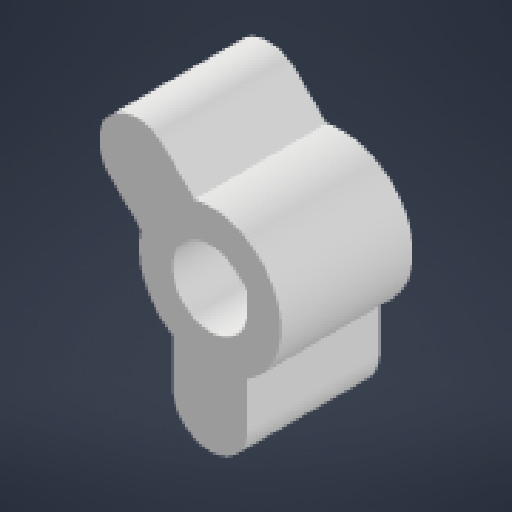
# Autodesk Inventor part: claw_joined_spacer
Saved by Autodesk Inventor 2026 (Build 300175000, 175)
## iProperties
Created: 2025-03-27
Part Number: claw_joined_spacer
Material: Generic
Document SubType Name: Modeling
Designer: paris
Density: 1 g/cm^3
Appearance: Default
Author: paris
Autodesk Inventor part; units mm, degrees
ref_plane "YZ Plane" through (0, 0, 0) normal (1, 0, 0) x (0, 1, 0)
ref_plane "XZ Plane" through (0, 0, 0) normal (0, 1, 0) x (-1, 0, 0)
ref_plane "XY Plane" through (0, 0, 0) normal (0, 0, 1) x (1, 0, 0)
sketch "Sketch1" plane through (0, 0, 0) normal (0, 0, 1) x (1, 0, 0)
  line L0 (-19.6493, 54.0192) -> (-19.6493, 51.5192) projected
  line L1 (-19.6493, 51.5192) -> (-17.1493, 50.3535) projected
  line L2 (-17.1493, 50.3535) -> (-17.1493, 47.8535) projected
  line L3 (-17.1493, 47.8535) -> (-19.6493, 46.6877) projected
  line L4 (-19.6493, 46.6877) -> (-19.6493, 44.1877) projected
  line L5 (-19.6493, 44.1877) -> (-17.1493, 43.0219) projected
  line L6 (-17.1493, 43.0219) -> (-17.1493, 40.5219) projected
  line L7 (-17.1493, 40.5219) -> (-19.6493, 39.3562) projected
  line L8 (-19.6493, 39.3562) -> (-19.6493, 36.8562) projected
  line L9 (-19.6493, 36.8562) -> (-17.1493, 35.6904) projected
  line L10 (-17.1493, 35.6904) -> (-17.1493, 33.1904) projected
  line L11 (-17.1493, 33.1904) -> (-19.6493, 32.0246) projected
  line L12 (-19.6493, 32.0246) -> (-19.6493, 29.5246) projected
  line L13 (-19.6493, 29.5246) -> (-17.1493, 28.3588) projected
  line L14 (-17.1493, 28.3588) -> (-17.1493, 27.685) projected
  arc A0 (-17.1493, 27.685) -> (-16.1428, 26.9802) centre (-16.3993, 27.685) ccw projected
  line L15 (-16.1428, 26.9802) -> (-10.6172, 28.9914) projected
  line L16 (-10.6172, 28.9914) -> (10.596, 7.7782) projected
  line L17 (10.596, 7.7782) -> (10.596, -7.2218) projected
  line L18 (10.596, -7.2218) -> (-10.6172, -28.435) projected
  line L19 (-10.6172, -28.435) -> (-10.6172, -58.435) projected
  line L20 (-10.6172, -58.435) -> (-0.6172, -58.435) projected
  line L21 (-0.6172, -58.435) -> (-0.6172, -33.435) projected
  line L22 (-0.6172, -33.435) -> (18.096, -14.7218) projected
  arc A1 (18.096, -14.7218) -> (19.6493, -10.9718) centre (14.346, -10.9718) ccw projected
  line L23 (19.6493, -10.9718) -> (19.6493, 11.5282) projected
  arc A2 (19.6493, 11.5282) -> (18.096, 15.2782) centre (14.346, 11.5282) ccw projected
  line L24 (18.096, 15.2782) -> (-10.6172, 43.9914) projected
  line L25 (-10.6172, 43.9914) -> (-15.6946, 57.9415) projected
  arc A3 (-15.6946, 57.9415) -> (-17.1493, 57.685) centre (-16.3993, 57.685) ccw projected
  line L26 (-17.1493, 57.685) -> (-17.1493, 55.185) projected
  line L27 (-17.1493, 55.185) -> (-19.6493, 54.0192) projected
  circle A4 centre (-5.6172, -50.935) radius 2 projected
  circle A5 centre (-5.6172, -35.935) radius 2 projected
  circle A6 centre (14.346, 11.5282) radius 2 projected
  circle A7 centre (14.346, -10.9718) radius 2 projected
  circle A8 centre (-10.6172, 36.4914) radius 2 projected
  circle A9 centre (14.346, 11.5282) radius 3.75
  line L28 (14.346, 11.5282) -> (14.346, 4.0282)
  line L29 (14.346, 11.5282) -> (9.0427, 16.8315)
  line L30 (14.346, 11.5282) -> (21.846, 11.5282) construction
  line L31 (11.8712, 16.8315) -> (16.346, 12.3566)
  line L32 (16.346, 12.3566) -> (16.346, 6.0282)
  line L33 (9.0427, 14.0031) -> (12.346, 10.6998)
  line L34 (12.346, 10.6998) -> (12.346, 6.0282)
  line L35 (14.346, 4.0282) -> (14.346, 4.0282)
  line L36 (9.0427, 16.8315) -> (9.0427, 16.8315)
  arc A10 (11.8712, 16.8315) -> (9.0427, 16.8315) centre (10.457, 15.4173) ccw
  arc A11 (9.0427, 16.8315) -> (9.0427, 14.0031) centre (10.457, 15.4173) ccw
  arc A12 (12.346, 6.0282) -> (14.346, 4.0282) centre (14.346, 6.0282) ccw
  arc A13 (14.346, 4.0282) -> (16.346, 6.0282) centre (14.346, 6.0282) ccw
  point P0 (0, 0)
  point P1 (15.7603, 12.9424)
  point P2 (16.346, 11.5282)
  point P3 (13.5172, 15.1855)
  point P4 (10.6888, 12.357)
  point P5 (12.346, 8.3561)
  point P6 (16.346, 8.3561)
  dimension "d0" = 7.5
  dimension "d2" = 7.5
  dimension "d3" = 135
  dimension "d4" = 2
  dimension "d5" = 2
  dimension "d6" = 7.5
  dimension "d7" = 2
  constraints: 18 end point, 8 point on circle, 8 tangent, 5 centre point, 3 equal radius, 2 horizontal, 2 midpoint, 1 coincident, 1 equal length, 1 perpendicular, 1 vertical, 2 other
  measures "d0" diameter of A9
  measures "d2" distance of L28.start L29.end
  measures "d3" angle of L30 L29
  measures "d4" distance between parallel lines of L29 L31
  measures "d5" distance between parallel lines of L29 L33
  measures "d6" distance of L28.start L28.end
  measures "d7" radius of A10
extrude "Extrusion1" add sketch "Sketch1" along normal blind 7 contours L32 A9 L28 A6 | A6 L31 L32 | L32 L31 A9 | A6 L29 A9 L31 | L28 A9 L34 L33 L29 A6 | L32 A13 L28 A9 | A9 L29 A10 L31 | L28 A12 L34 A9 | A9 L33 A11 L29 | A9 L33 L34
body "Solid1"
